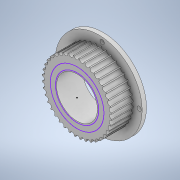
# Autodesk Inventor part: 051665019-12-1
Saved by Autodesk Inventor 2021 (Build 250183000, 183)
## iProperties
Created: 2020-05-14
Part Number: 051665019-12-1
Material: Generic
Document SubType Name: Modeling
Designer: figen
Density: 1 g/cm^3
Appearance: Default
Author: figen
Autodesk Inventor part; units mm, degrees
ref_plane "YZ Plane" through (0, 0, 0) normal (1, 0, 0) x (0, 1, 0)
ref_plane "XZ Plane" through (0, 0, 0) normal (0, 1, 0) x (-1, 0, 0)
ref_plane "XY Plane" through (0, 0, 0) normal (0, 0, 1) x (1, 0, 0)
sketch "Sketch1" plane through (0, 0, 0) normal (0, 0, 1) x (1, 0, 0)
  circle A0 centre (0, 0) radius 2540
  dimension "d0" = 5080
  constraints: 1 centre point, 1 coincident
  measures "d0" diameter of A0
extrude "Extrusion1" add sketch "Sketch1" along normal blind 254
sketch "Sketch2" plane through (0, 0, 254) normal (0, 0, 1) x (1, 0, 0)
  circle A0 centre (0, 0) radius 2032
  circle A1 centre (1460.7651, -1412.5117) radius 127
  circle A2 centre (1663.7462, -1166.6073) radius 127
  circle A3 centre (1825.7603, -891.9772) radius 127
  circle A4 centre (1942.8182, -595.3836) radius 127
  circle A5 centre (2012.0374, -284.1297) radius 127
  circle A6 centre (2031.7135, 34.1204) radius 127
  circle A7 centre (2001.3621, 351.5303) radius 127
  circle A8 centre (1921.7306, 660.2844) radius 127
  circle A9 centre (1794.7797, 952.7801) radius 127
  circle A10 centre (1623.6353, 1221.8152) radius 127
  circle A11 centre (1412.5117, 1460.7651) radius 127
  circle A12 centre (1166.6073, 1663.7462) radius 127
  circle A13 centre (891.9772, 1825.7603) radius 127
  circle A14 centre (595.3836, 1942.8182) radius 127
  circle A15 centre (284.1297, 2012.0374) radius 127
  circle A16 centre (-34.1204, 2031.7135) radius 127
  circle A17 centre (-351.5303, 2001.3621) radius 127
  circle A18 centre (-660.2844, 1921.7306) radius 127
  circle A19 centre (-952.7801, 1794.7797) radius 127
  circle A20 centre (-1221.8152, 1623.6353) radius 127
  circle A21 centre (-1460.7651, 1412.5117) radius 127
  circle A22 centre (-1663.7462, 1166.6073) radius 127
  circle A23 centre (-1825.7603, 891.9772) radius 127
  circle A24 centre (-1942.8182, 595.3836) radius 127
  circle A25 centre (-2012.0374, 284.1297) radius 127
  circle A26 centre (-2031.7135, -34.1204) radius 127
  circle A27 centre (-2001.3621, -351.5303) radius 127
  circle A28 centre (-1921.7306, -660.2844) radius 127
  circle A29 centre (-1794.7797, -952.7801) radius 127
  circle A30 centre (-1623.6353, -1221.8152) radius 127
  circle A31 centre (-1412.5117, -1460.7651) radius 127
  circle A32 centre (-1166.6073, -1663.7462) radius 127
  circle A33 centre (-891.9772, -1825.7603) radius 127
  circle A34 centre (-595.3836, -1942.8182) radius 127
  circle A35 centre (-284.1297, -2012.0374) radius 127
  circle A36 centre (34.1204, -2031.7135) radius 127
  circle A37 centre (351.5303, -2001.3621) radius 127
  circle A38 centre (660.2844, -1921.7306) radius 127
  circle A39 centre (952.7801, -1794.7797) radius 127
  circle A40 centre (1221.8152, -1623.6353) radius 127
  point P0 (1118.0012, -1696.7903)
  point P1 (1320.8565, -1544.138)
  point P2 (1369.6732, -1501.0061)
  point P3 (1546.151, -1318.4996)
  point P4 (1587.6194, -1268.2621)
  point P5 (1733.3741, -1060.3954)
  point P6 (1766.473, -1004.2893)
  point P7 (1877.9157, -776.1807)
  point P8 (1901.8303, -715.5876)
  point P9 (1976.2169, -472.8539)
  point P10 (1990.3582, -409.2657)
  point P11 (2025.857, -157.8839)
  point P12 (2029.8768, -92.8663)
  point P13 (2025.6138, 160.9738)
  point P14 (2019.4131, 225.8197)
  point P15 (1975.4933, 475.8678)
  point P16 (1959.2248, 538.9453)
  point P17 (1876.7296, 779.0443)
  point P18 (1850.7939, 838.8003)
  point P19 (1731.7546, 1063.0382)
  point P20 (1696.7903, 1118.0012)
  point P21 (1544.138, 1320.8565)
  point P22 (1501.0061, 1369.6732)
  point P23 (1318.4996, 1546.151)
  point P24 (1268.2621, 1587.6194)
  point P25 (1060.3954, 1733.3741)
  point P26 (1004.2893, 1766.473)
  point P27 (776.1807, 1877.9157)
  point P28 (715.5876, 1901.8303)
  point P29 (472.8539, 1976.2169)
  point P30 (409.2657, 1990.3582)
  point P31 (157.8839, 2025.857)
  point P32 (92.8663, 2029.8768)
  point P33 (-160.9738, 2025.6138)
  point P34 (-225.8197, 2019.4131)
  point P35 (-475.8678, 1975.4933)
  point P36 (-538.9453, 1959.2248)
  point P37 (-779.0443, 1876.7296)
  point P38 (-838.8003, 1850.7939)
  point P39 (-1063.0382, 1731.7546)
  point P40 (-1118.0012, 1696.7903)
  point P41 (-1320.8565, 1544.138)
  point P42 (-1369.6732, 1501.0061)
  point P43 (-1546.151, 1318.4996)
  point P44 (-1587.6194, 1268.2621)
  point P45 (-1733.3741, 1060.3954)
  point P46 (-1766.473, 1004.2893)
  point P47 (-1877.9157, 776.1807)
  point P48 (-1901.8303, 715.5876)
  point P49 (-1976.2169, 472.8539)
  point P50 (-1990.3582, 409.2657)
  point P51 (-2025.857, 157.8839)
  point P52 (-2029.8768, 92.8663)
  point P53 (-2025.6138, -160.9738)
  point P54 (-2019.4131, -225.8197)
  point P55 (-1975.4933, -475.8678)
  point P56 (-1959.2248, -538.9453)
  point P57 (-1876.7296, -779.0443)
  point P58 (-1850.7939, -838.8003)
  point P59 (-1731.7546, -1063.0382)
  point P60 (-1696.7903, -1118.0012)
  point P61 (-1544.138, -1320.8565)
  point P62 (-1501.0061, -1369.6732)
  point P63 (-1318.4996, -1546.151)
  point P64 (-1268.2621, -1587.6194)
  point P65 (-1060.3954, -1733.3741)
  point P66 (-1004.2893, -1766.473)
  point P67 (-776.1807, -1877.9157)
  point P68 (-715.5876, -1901.8303)
  point P69 (-472.8539, -1976.2169)
  point P70 (-409.2657, -1990.3582)
  point P71 (-157.8839, -2025.857)
  point P72 (-92.8663, -2029.8768)
  point P73 (160.9738, -2025.6138)
  point P74 (225.8197, -2019.4131)
  point P75 (475.8678, -1975.4933)
  point P76 (538.9453, -1959.2248)
  point P77 (779.0443, -1876.7296)
  point P78 (838.8003, -1850.7939)
  point P79 (1063.0382, -1731.7546)
  dimension "d3" = 4064
  dimension "d4" = 254
  dimension "d7" = 360
  constraints: 40 centre point, 1 coincident, 83 other
  measures "d4" diameter of A1
extrude "Extrusion2" add sketch "Sketch2" along normal blind 1270 contours A6 A0 A5 A4 A3 A2 A1 A40 A39 A38 A37 A36 A35 A34 A33 A32 A31 A30 A29 A28 A27 A26 A25 A24 A23 A22 A21 A20 A19 A18 A17 A16 A15 A14 A13 A12 A11 A10 A9 A8 A7
sketch "Sketch3" plane through (0, 0, 1524) normal (0, 0, 1) x (1, 0, 0)
  circle A0 centre (0, 0) radius 1193.2558
  constraints: 1 centre point, 1 coincident
extrude "Extrusion3" cut sketch "Sketch3" against normal blind 4257.675
sketch "Sketch4" plane through (0, 0, 1524) normal (0, 0, 1) x (1, 0, 0)
  circle A0 centre (0, 0) radius 1566.9494
  circle A1 centre (0, 0) radius 1262.4077
  constraints: 2 centre point, 2 coincident
sketch "Sketch5" plane through (0, 0, 254) normal (0, 0, 1) x (1, 0, 0)
  point P0 (0, 0)
  point P1 (2374.0298, -12.1015)
hole "Hole1" at (2374.0298, -12.1015, 254) direction (0, 0, -1) diameter 254 end through all
sketch "Sketch6" plane through (0, 0, 254) normal (0, 0, 1) x (1, 0, 0)
  point P0 (0, 0)
  point P1 (-330.2018, -2282.1198)
hole "Hole2" at (-330.2018, -2282.1198, 254) direction (0, 0, -1) diameter 254 end through all
sketch "Sketch7" plane through (0, 0, 254) normal (0, 0, 1) x (1, 0, 0)
  point P0 (0, 0)
  point P1 (209.5188, 2279.254)
hole "Hole3" at (209.5188, 2279.254, 254) direction (0, 0, -1) diameter 254 end through all
sketch "Sketch8" plane through (0, 0, 254) normal (0, 0, 1) x (1, 0, 0)
  point P0 (0, 0)
  point P1 (-2284.0066, 78.9189)
hole "Hole4" at (-2284.0066, 78.9189, 254) direction (0, 0, -1) diameter 254 end through all
body "Solid1"
